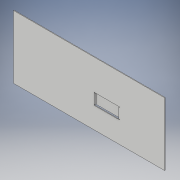
# Autodesk Inventor part: Ambutisare1
Saved by Autodesk Inventor 2019 (Build 230136000, 136)
## iProperties
Created: 2020-04-08
Part Number: Ambutisare1
Material: Generic
Document SubType Name: Sheet Metal
Designer: Gabriel
Density: 1 g/cm^3
Sheet Metal Rule: Default_mm
Appearance: Default
Author: Gabriel
Autodesk Inventor part; units mm, degrees
ref_plane "YZ Plane" through (0, 0, 0) normal (1, 0, 0) x (0, 1, 0)
ref_plane "XZ Plane" through (0, 0, 0) normal (0, 1, 0) x (-1, 0, 0)
ref_plane "XY Plane" through (0, 0, 0) normal (0, 0, 1) x (1, 0, 0)
sketch "Sketch1" plane through (0, 0, 0) normal (0, 0, 1) x (1, 0, 0)
  line L0 (-60.259, 41.2953) -> (59.741, 41.2953)
  line L1 (59.741, 41.2953) -> (59.741, -8.7047)
  line L2 (59.741, -8.7047) -> (-60.259, -8.7047)
  line L3 (-60.259, -8.7047) -> (-60.259, 41.2953)
  dimension "d0" = 120
  dimension "d1" = 50
  measures "d0" distance of L1.end L2.end
  measures "d1" distance of L0.end L1.end
extrude "Plate1" add sketch "Sketch1" along normal blind 0.5
sketch "Sketch2" plane through (0, 0, 0.5) normal (0, 0, 1) x (1, 0, 0)
  line L0 (3.7677, 16.6653) -> (23.7677, 16.6653)
  line L1 (23.7677, 16.6653) -> (23.7677, 8.6653)
  line L2 (23.7677, 8.6653) -> (3.7677, 8.6653)
  line L3 (3.7677, 8.6653) -> (3.7677, 16.6653)
  point P0 (13.7677, 12.6653)
  point P1 (13.7677, 12.6653)
  dimension "LG_G" = 20
  dimension "LT_G" = 8
  dimension "d5" = 10
  dimension "d6" = 4
  constraints: 8 end point, 2 parallel, 1 coincident, 1 horizontal, 1 perpendicular
  measures "LG_G" distance of L1.end L2.end
  measures "LT_G" distance of L0.end L1.end
  measures "d5" distance from line of L3 point (13.768, 12.665)
  measures "d6" distance from line of L2 point (13.768, 12.665)
extrude "Extrusion1" add sketch "Sketch2" against normal blind 1.5
sketch "Sketch3" plane through (0, 0, 0.5) normal (0, 0, 1) x (1, 0, 0)
  line L0 (3.7677, 16.6653) -> (23.7677, 16.6653) projected
  line L1 (3.7677, 8.6653) -> (3.7677, 16.6653) projected
  line L2 (23.7677, 8.6653) -> (3.7677, 8.6653) projected
  line L3 (23.7677, 16.6653) -> (23.7677, 8.6653) projected
  line L4 (4.2677, 16.6653) -> (23.2677, 16.6653)
  line L5 (23.2677, 16.6653) -> (23.2677, 8.6653)
  line L6 (23.2677, 8.6653) -> (4.2677, 8.6653)
  line L7 (4.2677, 8.6653) -> (4.2677, 16.6653)
  dimension "d9" = 0.5
  dimension "d10" = 0.5
  constraints: 8 end point, 2 collinear, 2 parallel, 1 horizontal, 1 perpendicular
  measures "d9" distance of L2.start L5.end
  measures "d10" distance of L0.start L4.start
extrude "Extrusion2" cut sketch "Sketch3" against normal blind 1 contours L0 L5 L2 L7
sketch "Sketch4" plane through (0, 0, 0.5) normal (0, 0, 1) x (1, 0, 0)
  line L0 (4.2677, 16.6653) -> (23.2677, 16.6653) projected
  line L1 (23.2677, 8.6653) -> (4.2677, 8.6653) projected
  line L2 (4.2677, 16.6653) -> (23.2677, 16.6653) projected
  line L3 (4.2677, 8.6653) -> (4.2677, 16.6653) projected
  line L4 (23.2677, 8.6653) -> (4.2677, 8.6653) projected
  line L5 (23.2677, 16.6653) -> (23.2677, 8.6653) projected
  line L6 (3.7677, 17.1653) -> (23.7677, 17.1653)
  line L7 (23.7677, 17.1653) -> (23.7677, 16.6653)
  line L8 (23.7677, 16.6653) -> (3.7677, 16.6653)
  line L9 (3.7677, 16.6653) -> (3.7677, 17.1653)
  line L10 (3.7677, 8.6653) -> (23.7677, 8.6653)
  line L11 (23.7677, 8.6653) -> (23.7677, 8.1653)
  line L12 (23.7677, 8.1653) -> (3.7677, 8.1653)
  line L13 (3.7677, 8.1653) -> (3.7677, 8.6653)
  dimension "d13" = 0.5
  dimension "d14" = 0.5
  dimension "d15" = 0.5
  dimension "d16" = 0.5
  constraints: 16 end point, 4 collinear, 4 parallel, 2 horizontal, 2 perpendicular
  measures "d13" distance of L8.end L6.start
  measures "d14" distance of L12.end L10.start
  measures "d15" distance of L10.start L1.end
  measures "d16" distance of L10.end L1.start
extrude "Cut1" cut sketch "Sketch4" against normal blind 0.5 contours L8 L9 L6 L7 L0 | L1 L10 L11 L12 L13
equation "\"d5\" = 0.5 * LG_G"
equation "\"d6\" = 0.5 * LT_G"
equation "\"d7\" = 3 * Thickness"
equation "\"d9\" = Thickness"
equation "\"d10\" = Thickness"
equation "\"d11\" = 2 * Thickness"
equation "\"d13\" = Thickness"
equation "\"d14\" = Thickness"
equation "\"d15\" = Thickness"
equation "\"d16\" = Thickness"
equation "\"d17\" = Thickness"
equation "\"d2\" = Thickness"
equation "\"BendRadius\" = Thickness"
equation "\"BendReliefWidth\" = Thickness"
equation "\"BendReliefDepth\" = 0.5 * Thickness"
equation "\"CornerReliefSize\" = 4 * Thickness"
equation "\"MinimumRemnant\" = 2 * Thickness"
equation "\"TransitionRadius\" = BendRadius"
equation "\"JacobiRadiusSize\" = BendRadius"
equation "\"GapSize\" = Thickness"
equation "\"Thickness\" = 0.5"
body "Solid1"
